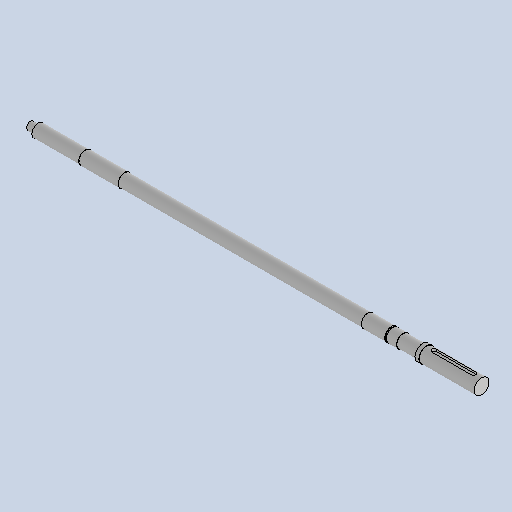
# Autodesk Inventor part: shaft 2
Saved by Autodesk Inventor 2025 (Build 290162010, 162A)
## iProperties
Created: 2024-09-24
Part Number: shaft 2
Material: Generic
Document SubType Name: Modeling
Designer: admin
Density: 1 g/cm^3
Appearance: Default
Stock Number: вал
Author: admin
Autodesk Inventor part; units mm, degrees
ref_plane "YZ Plane" through (0, 0, 0) normal (1, 0, 0) x (0, 1, 0)
ref_plane "XZ Plane" through (0, 0, 0) normal (0, 1, 0) x (-1, 0, 0)
sketch "Sketch1" plane through (0, 0, 0) normal (0, 0, 1) x (1, 0, 0)
  line L0 (0, 0) -> (115, 0)
  line L1 (115, 0) -> (115, 8.2)
  line L2 (115, 8.2) -> (-25, 8.2)
  line L3 (-25, 8.2) -> (-460, 8.2)
  line L4 (-460, 8.2) -> (-460, 0)
  line L5 (-460, 0) -> (0, 0)
  line L6 (-340, 8.2) -> (-340, 8.5)
  line L7 (-340, 8.5) -> (-390, 8.5)
  line L8 (-390, 8.5) -> (-390, 8.2)
  line L9 (15, 8.2) -> (15, 8.5)
  line L10 (15, 8.5) -> (-30, 8.5)
  line L11 (-30, 8.5) -> (-30, 8.2)
  line L12 (115, 8.2) -> (115, 9.5)
  line L13 (115, 9.5) -> (45, 9.5)
  line L14 (45, 9.5) -> (45, 8.2)
  line L15 (45, 9.5) -> (45, 10)
  line L16 (45, 10) -> (40, 10)
  line L17 (40, 10) -> (40, 8.2)
  line L18 (0, 8.5) -> (0, 7.5)
  line L19 (0, 7.5) -> (2, 7.5)
  line L20 (2, 7.5) -> (2, 8.5)
  line L21 (-460, 5) -> (-450, 5)
  line L22 (-450, 5) -> (-450, 8.2)
  dimension "d0" = 16.4
  dimension "d3" = 17
  dimension "d5" = 50
  dimension "d6" = 460
  dimension "d7" = 45
  dimension "d9" = 17
  dimension "d10" = 115
  dimension "d11" = 19
  dimension "d12" = 20
  dimension "d13" = 5
  dimension "d14" = 70
  dimension "d16" = 15
  dimension "d17" = 2
  dimension "d18" = 15
  dimension "d19" = 340
  dimension "d25" = 10
  dimension "d26" = 10
  constraints: 46 end point, 15 perpendicular, 13 point on line, 2 vertical, 1 collinear, 1 horizontal, 1 midpoint, 1 parallel
  measures "d0" diameter of L3 L5
  measures "d3" diameter of L7 L5
  measures "d5" distance of L6.end L7.end
  measures "d6" distance from line of L4 L0.start
  measures "d7" distance of L9.end L10.end
  measures "d9" diameter of L10 L0
  measures "d10" distance from line of L0.start L1
  measures "d11" diameter of L13 L0
  measures "d12" diameter of L16 L0
  measures "d13" distance of L15.end L16.end
  measures "d14" distance of L12.end L13.end
  measures "d16" distance from line of L0.start L9
  measures "d17" distance of L18.end L19.end
  measures "d18" diameter of L19 L0
  measures "d19" distance from line of L0.start L6
  measures "d25" diameter of L21 L5
  measures "d26" distance of L21.start L21.end
revolve "Revolution1" add sketch "Sketch1" angle 360 about axis through (0, 0, 0) along (1, 0, 0) contours L5 L4 L21 L22 L3 L2 L18 L19 L20 L1 L0 | L2 L14 L13 L12 | L2 L17 L16 L15 L14 | L2 L20 L10 L9 | L8 L7 L6 L3 | L2 L3 L11 L10 L18
ref_plane "Work Plane1" through (80, 0, 9.5) normal (0, 0, 1) x (1, 0, 0)
sketch "Sketch2" plane through (80, 0, 9.5) normal (0, 0, 1) x (1, 0, 0)
  line L0 (35, -9.5) -> (35, 9.5) projected
  line L1 (25, 0) -> (-25, 0) construction
  line L2 (25, 3) -> (-25, 3)
  line L3 (-25, -3) -> (25, -3)
  arc A0 (25, -3) -> (25, 3) centre (25, 0) ccw
  arc A1 (-25, 3) -> (-25, -3) centre (-25, 0) ccw
  point P0 (-80, 0)
  point P1 (0, 0)
  point P2 (35, 0)
  dimension "d20" = 6
  dimension "d21" = 50
  dimension "d22" = 35
  constraints: 8 end point, 4 point on circle, 4 tangent, 2 centre point, 2 midpoint, 1 horizontal, 1 horizontal alignment, 1 parallel
  measures "d20" diameter of A1
  measures "d21" distance of L1.start L1.end
  measures "d22" distance from line of L0 point (0, 0)
extrude "Extrusion1" cut sketch "Sketch2" against normal blind 3
body "Solid1"
